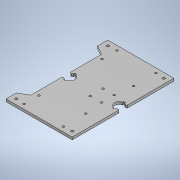
# Autodesk Inventor part: Base robot réduit
Saved by Autodesk Inventor 2022 (Build 260153000, 153)
## iProperties
Created: 2022-04-26
Part Number: Base robot réduit
Material: Générique
Document SubType Name: Modeling
Designer: victo
Density: 1 g/cm^3
Appearance: Transparent - Bleu
Author: victo
Autodesk Inventor part; units mm, degrees
ref_plane "YZ Plane" through (0, 0, 0) normal (1, 0, 0) x (0, 1, 0)
ref_plane "XZ Plane" through (0, 0, 0) normal (0, 1, 0) x (-1, 0, 0)
ref_plane "XY Plane" through (0, 0, 0) normal (0, 0, 1) x (1, 0, 0)
sketch "Esquisse1" plane through (0, 0, 0) normal (0, 1, 0) x (-1, 0, 0)
  line L0 (65, -100) -> (-65, -100)
  line L1 (-65, -100) -> (-65, 100)
  line L2 (-65, 100) -> (65, 100)
  line L3 (65, 100) -> (65, -100)
  line L4 (65, -100) -> (-65, 100) construction
  line L5 (-65, -100) -> (65, 100) construction
  line L6 (0, 100) -> (0, -100) construction
  line L7 (38.5, -91) -> (-38.5, -91) construction
  line L8 (-38.5, -91) -> (-38.5, -47) construction
  line L9 (-38.5, -47) -> (38.5, -47) construction
  line L10 (38.5, -47) -> (38.5, -91) construction
  line L11 (38.5, -91) -> (-38.5, -47) construction
  line L12 (-38.5, -91) -> (38.5, -47) construction
  circle A0 centre (38.5, -47) radius 2.1 construction
  circle A1 centre (38.5, -91) radius 2.1
  circle A2 centre (-38.5, -91) radius 2.1
  circle A3 centre (-38.5, -47) radius 2.1
  circle A4 centre (55, -90) radius 2.6
  line L13 (98.7177, 0) -> (-137.3062, 0) projected
  circle A5 centre (38.5, 91) radius 2.1
  circle A6 centre (-38.5, 91) radius 2.1
  circle A7 centre (-38.5, 47) radius 2.1
  circle A8 centre (55, 90) radius 2.6
  line L14 (-88.5885, -75) -> (-103.5885, -75)
  line L15 (-103.5885, -75) -> (-103.5885, 75)
  line L16 (-103.5885, 75) -> (-88.5885, 75)
  line L17 (-88.5885, 75) -> (-88.5885, -75)
  line L18 (-88.5885, -75) -> (-103.5885, 75) construction
  line L19 (-103.5885, -75) -> (-88.5885, 75) construction
  line L20 (-35, -12.5) -> (-13, -12.5) construction
  line L21 (-13, -12.5) -> (-13, 12.5) construction
  line L22 (-13, 12.5) -> (-35, 12.5) construction
  line L23 (-35, 12.5) -> (-35, -12.5) construction
  line L24 (-35, -12.5) -> (-13, 12.5) construction
  line L25 (-13, -12.5) -> (-35, 12.5) construction
  circle A9 centre (-55, -90) radius 2.6
  circle A10 centre (-55, 90) radius 2.6
  circle A11 centre (-13, 12.5) radius 2.1
  circle A12 centre (-13, -12.5) radius 2.1
  circle A13 centre (-35, -12.5) radius 2.1
  circle A14 centre (-35, 12.5) radius 2.1
  circle A15 centre (38.5, -62) radius 2.1
  circle A16 centre (38.5, 62) radius 2.1
  line L26 (65, -80) -> (47, -69.6077)
  line L27 (47, -69.6077) -> (47, 69.6077)
  line L28 (47, 69.6077) -> (65, 80)
  circle A17 centre (-57.1, 0) radius 9
  line L29 (-57.1, -9) -> (-57.1, -11.075) construction
  line L30 (-55.1, -11.075) -> (-59.1, -11.075)
  line L31 (-59.1, -11.075) -> (-59.1, -8.775)
  line L32 (-59.1, -8.775) -> (-55.1, -8.775) construction
  line L33 (-55.1, -8.775) -> (-55.1, -11.075)
  line L34 (-55.1, 11.075) -> (-59.1, 11.075)
  line L35 (-59.1, 11.075) -> (-59.1, 8.775)
  line L36 (-55.1, 8.775) -> (-55.1, 11.075)
  circle A18 centre (39.1, 0) radius 9
  line L37 (39.1, -9) -> (39.1, -11.075) construction
  line L38 (41.1, -11.075) -> (37.1, -11.075)
  line L39 (37.1, -11.075) -> (37.1, -8.775)
  line L40 (37.1, -8.775) -> (41.1, -8.775) construction
  line L41 (41.1, -8.775) -> (41.1, -11.075)
  line L42 (41.1, 11.075) -> (37.1, 11.075)
  line L43 (37.1, 11.075) -> (37.1, 8.775)
  line L44 (41.1, 8.775) -> (41.1, 11.075)
  point P0 (0, 0)
  point P1 (0, -69)
  point P2 (-96.0885, 0)
  point P3 (-24, 0)
  point P4 (-65, 4.3116)
  point P5 (-65, -4.3116)
  point P6 (47, -4.3116)
  point P7 (47, 4.3116)
  dimension "d0" = 65
  dimension "d1" = 130
  dimension "d2" = 200
  dimension "d3" = 77
  dimension "d4" = 44
  dimension "d6" = 4.2
  dimension "d7" = 16.5
  dimension "d8" = 5.2
  dimension "d9" = 10
  dimension "d10" = 10
  dimension "d11" = 9
  dimension "d12" = 15
  dimension "d13" = 150
  dimension "d15" = 25
  dimension "d16" = 22
  dimension "d17" = 30
  dimension "d18" = 16.5
  dimension "d21" = 10
  dimension "d22" = 10
  dimension "d23" = 4.2
  dimension "d26" = 15
  dimension "d27" = 10
  dimension "d28" = 10
  dimension "d29" = 60
  dimension "d30" = 18
  dimension "d31" = 60
  dimension "d37" = 7.9
  dimension "d38" = 18
  dimension "d39" = 4
  dimension "d40" = 2.3
  dimension "d41" = 7.9
  constraints: 88 end point, 19 centre point, 14 symmetric about line, 12 midpoint, 12 parallel, 10 point on line, 9 equal radius, 8 coincident, 7 perpendicular, 6 horizontal, 4 point on circle, 3 vertical, 2 equal length, 6 other
  measures "d0" distance between parallel lines of L6 L1
  measures "d1" distance of L0.start L0.end
  measures "d2" distance of L0.end L1.end
  measures "d3" distance of L8.end L9.end
  measures "d4" distance of L7.end L8.end
  measures "d6" diameter of A1
  measures "d7" distance from line of L10 A4.centre
  measures "d8" diameter of A4
  measures "d9" distance from line of L0 A4.centre
  measures "d10" distance from line of L3 A4.centre
  measures "d11" distance between parallel lines of L0 L7
  measures "d12" distance of L15.end L16.end
  measures "d13" distance of L14.end L15.end
  measures "d15" distance between parallel lines of L20 L22
  measures "d16" distance between parallel lines of L23 L21
  measures "d17" distance between parallel lines of L1 L23
  measures "d18" distance from line of A9.centre L8
  measures "d21" distance from line of L1 A9.centre
  measures "d22" distance from line of L0 A9.centre
  measures "d23" diameter of A11
  measures "d26" distance of L9.end A15.centre
  measures "d27" horizontal distance of L26.start A4.centre
  measures "d28" horizontal distance of A8.centre L28.end
  measures "d29" angle of L3 L28
  measures "d30" distance between parallel lines of L3 L27
  measures "d31" angle of L3 L26
  measures "d37" distance from line of L27 A18.centre
  measures "d38" diameter of A18
  measures "d39" distance of L38.start L38.end
  measures "d40" distance of L38.end L39.end
  measures "d41" distance from line of L1 A17.centre
extrude "Extrusion1" add sketch "Esquisse1" against normal blind 5 contours L0 L1 A17 L31 L30 L33 L13 A18 L39 L38 L41 L27 L26 L3 | L28 L27 A18 L44 L42 L43 L13 A17 L36 L34 L35 L1 L2 L3
fillet "Congé1" radius 2 4 edges at (65, -2.5, -4.3116) (65, -2.5, 4.3116) (-47, -2.5, -4.3116) (-47, -2.5, 4.3116)
